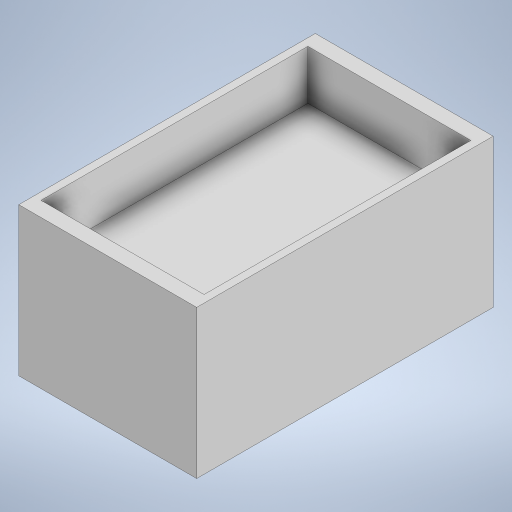
# Autodesk Inventor part: holder
Saved by Autodesk Inventor 2024 (Build 280153000, 153)
## iProperties
Created: 2025-01-06
Part Number: holder
Material: Generic
Document SubType Name: Modeling
Designer: Pavel
Density: 1 g/cm^3
Appearance: Default
Author: Pavel
Autodesk Inventor part; units mm, degrees
ref_plane "YZ Plane" through (0, 0, 0) normal (1, 0, 0) x (0, 1, 0)
ref_plane "XZ Plane" through (0, 0, 0) normal (0, 1, 0) x (-1, 0, 0)
ref_plane "XY Plane" through (0, 0, 0) normal (0, 0, 1) x (1, 0, 0)
sketch "Sketch1" plane through (0, 0, 0) normal (0, 1, 0) x (-1, 0, 0)
  line L0 (9, 15) -> (-9, 15)
  line L1 (-9, 15) -> (-9, -15)
  line L2 (-9, -15) -> (9, -15)
  line L3 (9, -15) -> (9, 15)
  point P0 (0, 0)
  dimension "d0" = 30
  dimension "d1" = 18
  dimension "d7" = 15
  dimension "d8" = 9
  constraints: 8 end point, 2 parallel, 1 horizontal, 1 perpendicular
  measures "d0" distance of L2.end L0.start
  measures "d1" distance of L0.start L0.end
  measures "d7" distance from line of L2 point (0, 0)
  measures "d8" distance from line of L3 point (0, 0)
extrude "Extrusion1" add sketch "Sketch1" along normal blind 15
sketch "Sketch2" plane through (0, 15, 0) normal (0, 1, 0) x (1, 0, 0)
  line L0 (-8.25, -13.5) -> (8.25, -13.5)
  line L1 (8.25, -13.5) -> (8.25, 13.5)
  line L2 (8.25, 13.5) -> (-8.25, 13.5)
  line L3 (-8.25, 13.5) -> (-8.25, -13.5)
  point P0 (0, 0)
  dimension "d4" = 27
  dimension "d5" = 16.5
  dimension "d6" = 13.5
  dimension "d9" = 8.25
  constraints: 8 end point, 2 parallel, 1 horizontal, 1 perpendicular
  measures "d4" distance of L2.end L0.start
  measures "d5" distance of L0.start L0.end
  measures "d6" distance from line of L2 point (0, 0)
  measures "d9" distance from line of L3 point (0, 0)
extrude "Extrusion2" cut sketch "Sketch2" against normal blind 5
sketch "Sketch3" plane through (0, 0, 0) normal (0, -1, 0) x (1, 0, 0)
  line L0 (3, 3) -> (-3, 3)
  line L1 (-3, 3) -> (-3, -3)
  line L2 (-3, -3) -> (3, -3)
  line L3 (3, -3) -> (3, 3)
  point P0 (0, 0)
  dimension "d12" = 6
  dimension "d13" = 6
  dimension "d14" = 3
  dimension "d15" = 3
  constraints: 8 end point, 2 parallel, 1 horizontal, 1 perpendicular
  measures "d12" distance of L2.end L0.start
  measures "d13" distance of L1.end L2.end
  measures "d14" distance from line of L2 point (0, 0)
  measures "d15" distance from line of L3 point (0, 0)
extrude "Extrusion3" cut sketch "Sketch3" against normal blind 8
equation "\"d7\" = 0.5 * d0"
equation "\"d8\" = 0.5 * d1"
equation "\"d6\" = 0.5 * d4"
equation "\"d9\" = 0.5 * d5"
equation "\"d14\" = 0.5 * d12"
equation "\"d15\" = 0.5 * d13"
body "Solid1"
